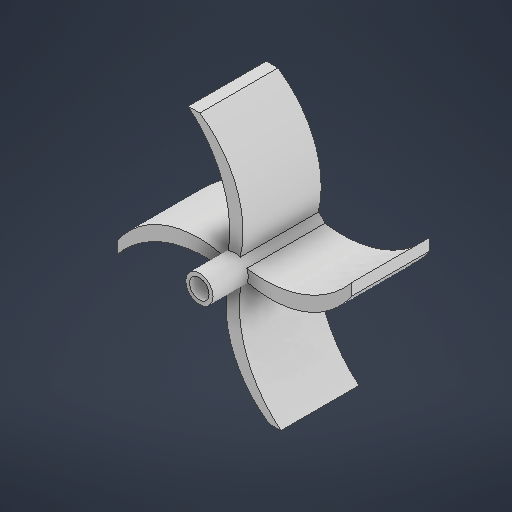
# Autodesk Inventor part: Naběračka
Saved by Autodesk Inventor 2026.1 (Build 301233000, 233)
## iProperties
Created: 2025-09-11
Part Number: Naběračka
Material: Všeobecné
Document SubType Name: Modeling
Designer: cerna
Density: 1 g/cm^3
Appearance: Výchozí
Author: cerna
Autodesk Inventor part; units mm, degrees
ref_plane "YZ Plane" through (0, 0, 0) normal (1, 0, 0) x (0, 1, 0)
ref_plane "XZ Plane" through (0, 0, 0) normal (0, 1, 0) x (-1, 0, 0)
ref_plane "XY Plane" through (0, 0, 0) normal (0, 0, 1) x (1, 0, 0)
sketch "Náčrt1" plane through (0, 0, 0) normal (0, 0, 1) x (1, 0, 0)
  line L0 (0, 4.9) -> (0, -4.9) projected
  line L1 (-4.9, 0) -> (4.9, 0) projected
  circle A0 centre (0, 0) radius 2.5
  circle A1 centre (0, 0) radius 3.5
  dimension "d0" = 5
  dimension "d1" = 7
  constraints: 2 centre point, 2 coincident
  measures "d0" diameter of A0
  measures "d1" diameter of A1
extrude "Vysunutí1" add sketch "Náčrt1" along normal blind 29 contours A1 L1 A0 L0 | L0 A0 L1 A1 | A1 L0 A0 L1 | L1 A0 L0 A1
sketch "Náčrt3" plane through (0, 0, 0) normal (0, 0, 1) x (1, 0, 0)
  circle A0 centre (0, 0) radius 3.5 projected
  line L0 (0, 44.2797) -> (0, -44.2797) projected
  line L1 (-44.2797, 0) -> (44.2797, 0) projected
  line L2 (-8.8727, 30) -> (-11.8727, 30)
  arc A1 (1.437, 3.1914) -> (-8.8727, 30) centre (-22.8177, 9.2506) ccw
  arc A2 (-1.5625, 3.1319) -> (-11.8727, 30) centre (-30.2246, 7.5455) ccw
  arc A3 (-3.1319, -1.5625) -> (-30, -11.8727) centre (-7.5455, -30.2246) ccw
  arc A4 (-3.1914, 1.437) -> (-30, -8.8727) centre (-9.2506, -22.8177) ccw
  line L3 (-30, -8.8727) -> (-30, -11.8727)
  arc A5 (1.5625, -3.1319) -> (11.8727, -30) centre (30.2246, -7.5455) ccw
  arc A6 (-1.437, -3.1914) -> (8.8727, -30) centre (22.8177, -9.2506) ccw
  line L4 (8.8727, -30) -> (11.8727, -30)
  arc A7 (3.1319, 1.5625) -> (30, 11.8727) centre (7.5455, 30.2246) ccw
  arc A8 (3.1914, -1.437) -> (30, 8.8727) centre (9.2506, 22.8177) ccw
  line L5 (30, 8.8727) -> (30, 11.8727)
  point P0 (-1.437, -3.1914)
  point P1 (1.5625, -3.1319)
  point P2 (-3.1914, 1.437)
  point P3 (-3.1319, -1.5625)
  point P4 (3.1319, 1.5625)
  point P5 (3.1914, -1.437)
  dimension "d4" = 25
  dimension "d5" = 29
  dimension "d6" = 3
  dimension "d7" = 3
  dimension "d8" = 30
  dimension "d11" = 360
  constraints: 18 point on circle, 8 centre point, 8 end point, 1 horizontal, 37 other
  measures "d4" radius of A1
  measures "d5" radius of A2
  measures "d6" distance of A0.start A0.end
  measures "d7" distance of L2.start L2.end
  measures "d8" distance between parallel lines of L1 L2
extrude "Vysunutí2" add sketch "Náčrt3" along normal blind 20 contours L1 A8 A0 | A0 A7 L5 A8 L1 | A0 L0 A1 | A5 L4 A6 L0 A0 | A0 A2 L2 A1 L0 | L0 A6 A0 | L1 A4 A0 | A0 A3 L3 A4 L1
